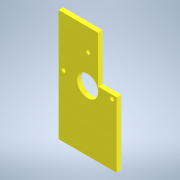
# Autodesk Inventor part: plateForHangingMechanism
Saved by Autodesk Inventor 2020.2 (Build 242310000, 310)
## iProperties
Created: 2020-01-06
Part Number: plateForHangingMechanism
Material: Aluminum 6061
Document SubType Name: Modeling
Designer: steele
Density: 2.7 g/cm^3
Appearance: Canary
Author: steele
Autodesk Inventor part; units mm, degrees
ref_plane "YZ Plane" through (0, 0, 0) normal (1, 0, 0) x (0, 1, 0)
ref_plane "XZ Plane" through (0, 0, 0) normal (0, 1, 0) x (-1, 0, 0)
ref_plane "XY Plane" through (0, 0, 0) normal (0, 0, 1) x (1, 0, 0)
sketch "Sketch1" plane through (0, 0, 0) normal (0, 0, 1) x (1, 0, 0)
  line L0 (-39.6875, -76.2) -> (39.6875, -76.2)
  line L1 (39.6875, -76.2) -> (39.6875, 76.2)
  line L2 (39.6875, 76.2) -> (-39.6875, 76.2)
  line L3 (-39.6875, 76.2) -> (-39.6875, -76.2)
  line L4 (-39.6875, -76.2) -> (39.6875, 76.2) construction
  line L5 (39.6875, -76.2) -> (-39.6875, 76.2) construction
  point P0 (0, 0)
  dimension "d0" = 79.375
  dimension "d1" = 152.4
  constraints: 12 end point, 2 midpoint, 2 parallel, 1 horizontal, 1 perpendicular
  measures "d0" distance of L0.start L0.end
  measures "d1" distance of L1.end L0.end
extrude "Extrusion1" add sketch "Sketch1" against normal blind 6.35
sketch "Sketch2" plane through (0, 0, 0) normal (0, 0, 1) x (1, 0, 0)
  circle A0 centre (0, 6.35) radius 14.4145
  line L0 (39.6875, 76.2) -> (-39.6875, 76.2) projected
  point P0 (0, 0)
  dimension "bearingDiameter" = 28.829
  dimension "d5" = 69.85
  constraints: 1 centre point
  measures "bearingDiameter" diameter of A0
  measures "d5" distance from line of A0.centre L0
extrude "Extrusion2" cut sketch "Sketch2" against normal through all
sketch "Sketch8" plane through (0, 0, 0) normal (0, 0, 1) x (1, 0, 0)
  line L0 (-39.6875, 76.2) -> (39.6875, 76.2) projected
  line L1 (39.6875, 76.2) -> (14.2875, 76.2)
  line L2 (14.2875, 76.2) -> (14.2875, 12.7)
  line L3 (14.2875, 12.7) -> (39.6875, 12.7)
  line L4 (39.6875, 12.7) -> (39.6875, 76.2)
  point P0 (0, 0)
  dimension "d43" = 25.4
  dimension "d44" = 63.5
  constraints: 8 end point, 2 parallel, 1 horizontal, 1 perpendicular
  measures "d43" distance of L3.end L2.end
  measures "d44" distance of L2.end L1.end
extrude "Extrusion3" cut sketch "Sketch8" against normal through all
sketch "Sketch9" plane through (0, 0, -6.35) normal (0, 0, -1) x (-1, 0, 0)
  point P0 (-0.5774, 46.336)
  point P1 (32.9749, 8.3263)
  point P2 (-33.0182, 7.3734)
hole "Hole8" at (0.5774, 46.336, -6.35) at (-32.9749, 8.3263, -6.35) at (33.0182, 7.3734, -6.35) direction (0, 0, 1) diameter 5.1054 depth 6.35
body "Solid1"
